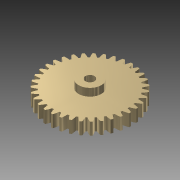
# Autodesk Inventor part: engrane4
Saved by Autodesk Inventor 2014 SP1 (Build 180222100, 222)
## iProperties
Created: 2017-09-24
Part Number: engrane4
Material: Generic
Document SubType Name: Modeling
Designer: Vivi
Density: 1 g/cm^3
Appearance: Default
Author: Vivi
Autodesk Inventor part; units mm, degrees
ref_plane "YZ Plane" through (0, 0, 0) normal (1, 0, 0) x (0, 1, 0)
ref_plane "XZ Plane" through (0, 0, 0) normal (0, 1, 0) x (-1, 0, 0)
ref_plane "XY Plane" through (0, 0, 0) normal (0, 0, 1) x (1, 0, 0)
sketch "Sketch1" plane through (0, 0, 0) normal (0, 0, 1) x (1, 0, 0)
  circle A0 centre (0, 0) radius 1.75
  arc A1 (5.9558, 23.6362) -> (5.5664, 27.186) centre (-9.9956, 23.6825) ccw
  arc A2 (5.5664, 27.186) -> (4.3411, 27.4084) centre (0, 0) ccw
  arc A3 (4.3411, 27.4084) -> (2.7291, 24.2217) centre (17.6796, 18.6602) ccw
  arc A4 (2.7291, 24.2217) -> (1.6397, 24.3198) centre (0, 0) ccw
  arc A5 (1.6397, 24.3198) -> (0.6227, 27.743) centre (-14.0636, 21.5171) ccw
  arc A6 (0.6227, 27.743) -> (-0.6227, 27.743) centre (0, 0) ccw
  arc A7 (-0.6227, 27.743) -> (-1.6397, 24.3198) centre (14.0636, 21.5171) ccw
  arc A8 (-1.6397, 24.3198) -> (-2.7291, 24.2217) centre (0, 0) ccw
  arc A9 (-2.7291, 24.2217) -> (-4.3411, 27.4084) centre (-17.6796, 18.6602) ccw
  arc A10 (-4.3411, 27.4084) -> (-5.5664, 27.186) centre (0, 0) ccw
  arc A11 (-5.5664, 27.186) -> (-5.9558, 23.6362) centre (9.9956, 23.6825) ccw
  arc A12 (-5.9558, 23.6362) -> (-7.0102, 23.3452) centre (0, 0) ccw
  arc A13 (-7.0102, 23.3452) -> (-9.1652, 26.1928) centre (-20.7274, 15.2035) ccw
  arc A14 (-9.1652, 26.1928) -> (-10.3311, 25.7552) centre (0, 0) ccw
  arc A15 (-10.3311, 25.7552) -> (-10.0805, 22.1929) centre (5.6063, 25.0867) ccw
  arc A16 (-10.0805, 22.1929) -> (-11.066, 21.7183) centre (0, 0) ccw
  arc A17 (-11.066, 21.7183) -> (-13.6949, 24.1353) centre (-23.109, 11.2581) ccw
  arc A18 (-13.6949, 24.1353) -> (-14.7639, 23.4966) centre (0, 0) ccw
  arc A19 (-14.7639, 23.4966) -> (-13.8812, 20.0363) centre (1.0368, 25.6845) ccw
  arc A20 (-13.8812, 20.0363) -> (-14.7661, 19.3933) centre (0, 0) ccw
  arc A21 (-14.7661, 19.3933) -> (-17.7843, 21.3021) centre (-24.7478, 6.9509) ccw
  arc A22 (-17.7843, 21.3021) -> (-18.7221, 20.4828) centre (0, 0) ccw
  arc A23 (-18.7221, 20.4828) -> (-17.2357, 17.2357) centre (-3.566, 25.4569) ccw
  arc A24 (-17.2357, 17.2357) -> (-17.9917, 16.4451) centre (0, 0) ccw
  arc A25 (-17.9917, 16.4451) -> (-21.3021, 17.7843) centre (-25.5913, 2.4203) ccw
  arc A26 (-21.3021, 17.7843) -> (-22.0786, 16.8107) centre (0, 0) ccw
  arc A27 (-22.0786, 16.8107) -> (-20.0363, 13.8812) centre (-8.0542, 24.4111) ccw
  arc A28 (-20.0363, 13.8812) -> (-20.6389, 12.9683) centre (0, 0) ccw
  arc A29 (-20.6389, 12.9683) -> (-24.1353, 13.6949) centre (-25.6122, -2.1881) ccw
  arc A30 (-24.1353, 13.6949) -> (-24.7254, 12.5982) centre (0, 0) ccw
  arc A31 (-24.7254, 12.5982) -> (-22.1929, 10.0805) centre (-12.2836, 22.5806) ccw
  arc A32 (-22.1929, 10.0805) -> (-22.6228, 9.0747) centre (0, 0) ccw
  arc A33 (-22.6228, 9.0747) -> (-26.1928, 9.1652) centre (-24.8099, -6.7261) ccw
  arc A34 (-26.1928, 9.1652) -> (-26.5776, 7.9809) centre (0, 0) ccw
  arc A35 (-26.5776, 7.9809) -> (-23.6362, 5.9558) centre (-16.1181, 20.0244) ccw
  arc A36 (-23.6362, 5.9558) -> (-23.8796, 4.8894) centre (0, 0) ccw
  arc A37 (-23.8796, 4.8894) -> (-27.4084, 4.3411) centre (-23.2102, -11.048) ccw
  arc A38 (-27.4084, 4.3411) -> (-27.5755, 3.107) centre (0, 0) ccw
  arc A39 (-27.5755, 3.107) -> (-24.3198, 1.6397) centre (-19.4346, 16.8246) ccw
  arc A40 (-24.3198, 1.6397) -> (-24.3689, 0.5469) centre (0, 0) ccw
  arc A41 (-24.3689, 0.5469) -> (-27.743, -0.6227) centre (-20.8645, -15.0148) ccw
  arc A42 (-27.743, -0.6227) -> (-27.6871, -1.8667) centre (0, 0) ccw
  arc A43 (-27.6871, -1.8667) -> (-24.2217, -2.7291) centre (-22.1264, 13.0841) ccw
  arc A44 (-24.2217, -2.7291) -> (-24.0749, -3.8131) centre (0, 0) ccw
  arc A45 (-24.0749, -3.8131) -> (-27.186, -5.5664) centre (-17.8482, -18.499) ccw
  arc A46 (-27.186, -5.5664) -> (-26.9089, -6.7804) centre (0, 0) ccw
  arc A47 (-26.9089, -6.7804) -> (-23.3452, -7.0102) centre (-24.1071, 8.923) ccw
  arc A48 (-23.3452, -7.0102) -> (-23.0072, -8.0506) centre (0, 0) ccw
  arc A49 (-23.0072, -8.0506) -> (-25.7552, -10.3311) centre (-14.2582, -21.3886) ccw
  arc A50 (-25.7552, -10.3311) -> (-25.2658, -11.4762) centre (0, 0) ccw
  arc A51 (-25.2658, -11.4762) -> (-21.7183, -11.066) centre (-25.3129, 4.4751) ccw
  arc A52 (-21.7183, -11.066) -> (-21.1999, -12.0293) centre (0, 0) ccw
  arc A53 (-21.1999, -12.0293) -> (-23.4966, -14.7639) centre (-10.21, -23.5908) ccw
  arc A54 (-23.4966, -14.7639) -> (-22.8106, -15.8032) centre (0, 0) ccw
  arc A55 (-22.8106, -15.8032) -> (-19.3933, -14.7661) centre (-25.7052, -0.1166) ccw
  arc A56 (-19.3933, -14.7661) -> (-18.7113, -15.6213) centre (0, 0) ccw
  arc A57 (-18.7113, -15.6213) -> (-20.4828, -18.7221) centre (-5.8336, -25.0348) ccw
  arc A58 (-20.4828, -18.7221) -> (-19.6222, -19.6222) centre (0, 0) ccw
  arc A59 (-19.6222, -19.6222) -> (-16.4451, -17.9917) centre (-25.2713, -4.7046) ccw
  arc A60 (-16.4451, -17.9917) -> (-15.6213, -18.7113) centre (0, 0) ccw
  arc A61 (-15.6213, -18.7113) -> (-16.8107, -22.0786) centre (-1.2697, -25.6741) ccw
  arc A62 (-16.8107, -22.0786) -> (-15.8032, -22.8106) centre (0, 0) ccw
  arc A63 (-15.8032, -22.8106) -> (-12.9683, -20.6389) centre (-24.0251, -9.1413) ccw
  arc A64 (-12.9683, -20.6389) -> (-12.0293, -21.1999) centre (0, 0) ccw
  arc A65 (-12.0293, -21.1999) -> (-12.5982, -24.7254) centre (3.335, -25.4882) ccw
  arc A66 (-12.5982, -24.7254) -> (-11.4762, -25.2658) centre (0, 0) ccw
  arc A67 (-11.4762, -25.2658) -> (-9.0747, -22.6228) centre (-22.0068, -13.2843) ccw
  arc A68 (-9.0747, -22.6228) -> (-8.0506, -23.0072) centre (0, 0) ccw
  arc A69 (-8.0506, -23.0072) -> (-7.9809, -26.5776) centre (7.8325, -24.4831) ccw
  arc A70 (-7.9809, -26.5776) -> (-6.7804, -26.9089) centre (0, 0) ccw
  arc A71 (-6.7804, -26.9089) -> (-4.8894, -23.8796) centre (-19.2811, -17.0002) ccw
  arc A72 (-4.8894, -23.8796) -> (-3.8131, -24.0749) centre (0, 0) ccw
  arc A73 (-3.8131, -24.0749) -> (-3.107, -27.5755) centre (12.0782, -22.6911) ccw
  arc A74 (-3.107, -27.5755) -> (-1.8667, -27.6871) centre (0, 0) ccw
  arc A75 (-1.8667, -27.6871) -> (-0.5469, -24.3689) centre (-15.9358, -20.1698) ccw
  arc A76 (-0.5469, -24.3689) -> (0.5469, -24.3689) centre (0, 0) ccw
  arc A77 (0.5469, -24.3689) -> (1.8667, -27.6871) centre (15.9358, -20.1698) ccw
  arc A78 (1.8667, -27.6871) -> (3.107, -27.5755) centre (0, 0) ccw
  arc A79 (3.107, -27.5755) -> (3.8131, -24.0749) centre (-12.0782, -22.6911) ccw
  arc A80 (3.8131, -24.0749) -> (4.8894, -23.8796) centre (0, 0) ccw
  arc A81 (4.8894, -23.8796) -> (6.7804, -26.9089) centre (19.2811, -17.0002) ccw
  arc A82 (6.7804, -26.9089) -> (7.9809, -26.5776) centre (0, 0) ccw
  arc A83 (7.9809, -26.5776) -> (8.0506, -23.0072) centre (-7.8325, -24.4831) ccw
  arc A84 (8.0506, -23.0072) -> (9.0747, -22.6228) centre (0, 0) ccw
  arc A85 (9.0747, -22.6228) -> (11.4762, -25.2658) centre (22.0068, -13.2843) ccw
  arc A86 (11.4762, -25.2658) -> (12.5982, -24.7254) centre (0, 0) ccw
  arc A87 (12.5982, -24.7254) -> (12.0293, -21.1999) centre (-3.335, -25.4882) ccw
  arc A88 (12.0293, -21.1999) -> (12.9683, -20.6389) centre (0, 0) ccw
  arc A89 (12.9683, -20.6389) -> (15.8032, -22.8106) centre (24.0251, -9.1413) ccw
  arc A90 (15.8032, -22.8106) -> (16.8107, -22.0786) centre (0, 0) ccw
  arc A91 (16.8107, -22.0786) -> (15.6213, -18.7113) centre (1.2697, -25.6741) ccw
  arc A92 (15.6213, -18.7113) -> (16.4451, -17.9917) centre (0, 0) ccw
  arc A93 (16.4451, -17.9917) -> (19.6222, -19.6222) centre (25.2713, -4.7046) ccw
  arc A94 (19.6222, -19.6222) -> (20.4828, -18.7221) centre (0, 0) ccw
  arc A95 (20.4828, -18.7221) -> (18.7113, -15.6213) centre (5.8336, -25.0348) ccw
  arc A96 (18.7113, -15.6213) -> (19.3933, -14.7661) centre (0, 0) ccw
  arc A97 (19.3933, -14.7661) -> (22.8106, -15.8032) centre (25.7052, -0.1166) ccw
  arc A98 (22.8106, -15.8032) -> (23.4966, -14.7639) centre (0, 0) ccw
  arc A99 (23.4966, -14.7639) -> (21.1999, -12.0293) centre (10.21, -23.5908) ccw
  arc A100 (21.1999, -12.0293) -> (21.7183, -11.066) centre (0, 0) ccw
  arc A101 (21.7183, -11.066) -> (25.2658, -11.4762) centre (25.3129, 4.4751) ccw
  arc A102 (25.2658, -11.4762) -> (25.7552, -10.3311) centre (0, 0) ccw
  arc A103 (25.7552, -10.3311) -> (23.0072, -8.0506) centre (14.2582, -21.3886) ccw
  arc A104 (23.0072, -8.0506) -> (23.3452, -7.0102) centre (0, 0) ccw
  arc A105 (23.3452, -7.0102) -> (26.9089, -6.7804) centre (24.1071, 8.923) ccw
  arc A106 (26.9089, -6.7804) -> (27.186, -5.5664) centre (0, 0) ccw
  arc A107 (27.186, -5.5664) -> (24.0749, -3.8131) centre (17.8482, -18.499) ccw
  arc A108 (24.0749, -3.8131) -> (24.2217, -2.7291) centre (0, 0) ccw
  arc A109 (24.2217, -2.7291) -> (27.6871, -1.8667) centre (22.1264, 13.0841) ccw
  arc A110 (27.6871, -1.8667) -> (27.743, -0.6227) centre (0, 0) ccw
  arc A111 (27.743, -0.6227) -> (24.3689, 0.5469) centre (20.8645, -15.0148) ccw
  arc A112 (24.3689, 0.5469) -> (24.3198, 1.6397) centre (0, 0) ccw
  arc A113 (24.3198, 1.6397) -> (27.5755, 3.107) centre (19.4346, 16.8246) ccw
  arc A114 (27.5755, 3.107) -> (27.4084, 4.3411) centre (0, 0) ccw
  arc A115 (27.4084, 4.3411) -> (23.8796, 4.8894) centre (23.2102, -11.048) ccw
  arc A116 (23.8796, 4.8894) -> (23.6362, 5.9558) centre (0, 0) ccw
  arc A117 (23.6362, 5.9558) -> (26.5776, 7.9809) centre (16.1181, 20.0244) ccw
  arc A118 (26.5776, 7.9809) -> (26.1928, 9.1652) centre (0, 0) ccw
  arc A119 (26.1928, 9.1652) -> (22.6228, 9.0747) centre (24.8099, -6.7261) ccw
  arc A120 (22.6228, 9.0747) -> (22.1929, 10.0805) centre (0, 0) ccw
  arc A121 (22.1929, 10.0805) -> (24.7254, 12.5982) centre (12.2836, 22.5806) ccw
  arc A122 (24.7254, 12.5982) -> (24.1353, 13.6949) centre (0, 0) ccw
  arc A123 (24.1353, 13.6949) -> (20.6389, 12.9683) centre (25.6122, -2.1881) ccw
  arc A124 (20.6389, 12.9683) -> (20.0363, 13.8812) centre (0, 0) ccw
  arc A125 (20.0363, 13.8812) -> (22.0786, 16.8107) centre (8.0542, 24.4111) ccw
  arc A126 (22.0786, 16.8107) -> (21.3021, 17.7843) centre (0, 0) ccw
  arc A127 (21.3021, 17.7843) -> (17.9917, 16.4451) centre (25.5913, 2.4203) ccw
  arc A128 (17.9917, 16.4451) -> (17.2357, 17.2357) centre (0, 0) ccw
  arc A129 (17.2357, 17.2357) -> (18.7221, 20.4828) centre (3.566, 25.4569) ccw
  arc A130 (18.7221, 20.4828) -> (17.7843, 21.3021) centre (0, 0) ccw
  arc A131 (17.7843, 21.3021) -> (14.7661, 19.3933) centre (24.7478, 6.9509) ccw
  arc A132 (14.7661, 19.3933) -> (13.8812, 20.0363) centre (0, 0) ccw
  arc A133 (13.8812, 20.0363) -> (14.7639, 23.4966) centre (-1.0368, 25.6845) ccw
  arc A134 (14.7639, 23.4966) -> (13.6949, 24.1353) centre (0, 0) ccw
  arc A135 (13.6949, 24.1353) -> (11.066, 21.7183) centre (23.109, 11.2581) ccw
  arc A136 (11.066, 21.7183) -> (10.0805, 22.1929) centre (0, 0) ccw
  arc A137 (10.0805, 22.1929) -> (10.3311, 25.7552) centre (-5.6063, 25.0867) ccw
  arc A138 (10.3311, 25.7552) -> (9.1652, 26.1928) centre (0, 0) ccw
  arc A139 (9.1652, 26.1928) -> (7.0102, 23.3452) centre (20.7274, 15.2035) ccw
  arc A140 (7.0102, 23.3452) -> (5.9558, 23.6362) centre (0, 0) ccw
  constraints: 280 point on circle, 141 centre point
extrude "Extrusion1" add sketch "Sketch1" along normal blind 8
sketch "Sketch2" plane through (0, 0, 8) normal (0, 0, 1) x (1, 0, 0)
  circle A0 centre (0, 0) radius 1.75 projected
  arc A1 (-10.0805, 22.1929) -> (-11.066, 21.7183) centre (0, 0) ccw projected
  circle A2 centre (0, 0) radius 7.5
  dimension "d2" = 15
  constraints: 1 centre point, 1 coincident
  measures "d2" diameter of A2
extrude "Extrusion2" add sketch "Sketch2" along normal blind 5
sketch "Sketch3" plane through (0, 0, 13) normal (0, 0, 1) x (1, 0, 0)
  circle A0 centre (0, 0) radius 1.75 projected
  circle A1 centre (0, 0) radius 7.5 projected
  circle A2 centre (0, 0) radius 3
  dimension "d5" = 6
  constraints: 1 centre point, 1 coincident
  measures "d5" diameter of A2
extrude "Extrusion3" cut sketch "Sketch3" against normal blind 5 contours A2
body "Solid1"
